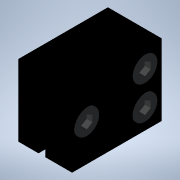
# Autodesk Inventor part: SCHUNK-5503506 Halter fuer NHS KL03
Saved by Autodesk Inventor 2021 (Build 250183000, 183)
## iProperties
Created: 2025-07-30
Part Number: SCHUNK-5503506 Halter fuer NHS KL03
Material: Generic
Catalog Web Link: www.cadenas.de
Description: KLH-bracket
Vendor: SCHUNK
Document SubType Name: Modeling
Designer: psAdmin
Manufacturer: SCHUNK
Mass: 2.81228 g
Surface Area: 23.0408 cm^2
Volume: 2.81228 cm^3
Density: 1 g/cm^3
Appearance: PSOLRGB-35-35-35
Category: PARTsolutions
Company: SCHUNK
Title: SCHUNK-5503506 Halter fuer NHS KL03.
Author: Cadenas PARTsolutions
Comments: bracket
PSOL_IDENT_0: {$CADENAS_DATA/23d-libs/schunk/greifsysteme/greifmodule/greifmodule_pneumatisch/3_finger_zentrischgr
PSOL_IDENT_1: eifer/3_finger_universalgreifer/jgz/jgz_klh.prj},208 {VTYP=3D},{NB=SCHUNK-5503506 Halter fuer NHS KL
PSOL_IDENT_2: 03},{LINA=SCHUNK-5503506 Halter fuer NHS KL03.},{NN=KLH},{DATE=18.12.2024 09:59:27},{GEOMDATE=23.09.
PSOL_IDENT_3: 2021 06:23:09},{VERSION=},{LINEID=10},{WBVAR=},{WBNUMERIC=}  {NB=SCHUNK-5503506 Halter fuer NHS KL03
PSOL_IDENT_4: },{LINA=SCHUNK-5503506 Halter fuer NHS KL03.},{KT=Halter fuer NHS KL03},{IDNR=5503506},{TYP=Halter f
PSOL_IDENT_5: uer NHS KL03},{TYP1=1.000},{L1=2.000},{B=12.000},{T=16.000},{CNSCTN=84799070}
NB: SCHUNK-5503506 Halter fuer NHS KL03
NN: KLH
NT: bracket
NBSYN: SCHUNK-$IDNR. $TYP.
LINA: SCHUNK-5503506 Halter fuer NHS KL03.
CATALOG: SCHUNK
IDNR: 5503506
TYP: Halter fuer NHS KL03
TYP1: 1
L1: 2
B: 12
T: 16
CNSCTN: 84799070
SUPPLIER: SCHUNK
ARTICLENO: SCHUNK-5503506 Halter fuer NHS KL03
BOMINFO: SCHUNK-5503506 Halter fuer NHS KL03.
CREATOR: CADENAS GmbH
Autodesk Inventor part; units mm, degrees
sketch "Skizze_1" plane through (0, 0, 0) normal (0, 1, 0) x (-1, 0, 0)
  line L0 (0, 10) -> (-4.5, 10)
  line L1 (-4.5, 10) -> (-4.5, 3.9686)
  arc A0 (-6, 3.873) -> (-4.5, 3.9686) centre (-5, 0) ccw
  line L2 (-6, 3.873) -> (-6, 10)
  line L3 (-6, 10) -> (-12, 10)
  line L4 (-12, 10) -> (-12, -10)
  line L5 (-12, -10) -> (0, -10)
  line L6 (0, -10) -> (0, 10)
  constraints: 14 end point, 2 point on circle, 1 centre point
extrude "Extrusion1" add sketch "Skizze_1" along normal blind 16
sketch "Sketch2" plane through (12, 0, 10) normal (1, 0, 0) x (0, 0, -1)
  point P0 (16.5, 4.25)
hole "Hole1" at (12, 4.25, -6.5) direction (-1, 0, 0) diameter 6 depth 3.2
sketch "Sketch3" plane through (12, 0, 10) normal (1, 0, 0) x (0, 0, -1)
  point P0 (16.5, 11.75)
hole "Hole2" at (12, 11.75, -6.5) direction (-1, 0, 0) diameter 6 depth 3.2
sketch "Skizze_5" plane through (8.8, 4.25, -6.5) normal (1, 0, 0) x (0, 0, -1)
  circle A0 centre (0, 0) radius 2.75
  constraints: 1 centre point
extrude "Extrusion2" add sketch "Skizze_5" along normal blind 3
sketch "Skizze_6" plane through (11.8, 4.25, -6.5) normal (1, 0, 0) x (0, 0, -1)
  line L0 (-1.25, -0.7217) -> (0, -1.4434)
  line L1 (0, -1.4434) -> (1.25, -0.7217)
  line L2 (1.25, -0.7217) -> (1.25, 0.7217)
  line L3 (1.25, 0.7217) -> (0, 1.4434)
  line L4 (0, 1.4434) -> (-1.25, 0.7217)
  line L5 (-1.25, 0.7217) -> (-1.25, -0.7217)
  constraints: 12 end point
extrude "Extrusion3" cut sketch "Skizze_6" against normal blind 1.3
sketch "Skizze_4" plane through (8.8, 11.75, -6.5) normal (1, 0, 0) x (0, 0, -1)
  circle A0 centre (0, 0) radius 2.75
  constraints: 1 centre point
extrude "Extrusion4" add sketch "Skizze_4" along normal blind 3
sketch "Skizze_7" plane through (11.8, 11.75, -6.5) normal (1, 0, 0) x (0, 0, -1)
  line L0 (-1.25, -0.7217) -> (0, -1.4434)
  line L1 (0, -1.4434) -> (1.25, -0.7217)
  line L2 (1.25, -0.7217) -> (1.25, 0.7217)
  line L3 (1.25, 0.7217) -> (0, 1.4434)
  line L4 (0, 1.4434) -> (-1.25, 0.7217)
  line L5 (-1.25, 0.7217) -> (-1.25, -0.7217)
  constraints: 12 end point
extrude "Extrusion5" cut sketch "Skizze_7" against normal blind 1.3
sketch "Sketch8" plane through (12, 0, 10) normal (1, 0, 0) x (0, 0, -1)
  point P0 (3.5, 8)
hole "Hole3" at (12, 8, 6.5) direction (-1, 0, 0) diameter 6 depth 3.2
sketch "Skizze_12" plane through (8.8, 8, 6.5) normal (1, 0, 0) x (0, 0, -1)
  circle A0 centre (0, 0) radius 2.75
  constraints: 1 centre point
extrude "Extrusion6" add sketch "Skizze_12" along normal blind 3
sketch "Skizze_13" plane through (11.8, 8, 6.5) normal (1, 0, 0) x (0, 0, -1)
  line L0 (-1.25, -0.7217) -> (0, -1.4434)
  line L1 (0, -1.4434) -> (1.25, -0.7217)
  line L2 (1.25, -0.7217) -> (1.25, 0.7217)
  line L3 (1.25, 0.7217) -> (0, 1.4434)
  line L4 (0, 1.4434) -> (-1.25, 0.7217)
  line L5 (-1.25, 0.7217) -> (-1.25, -0.7217)
  constraints: 12 end point
extrude "Extrusion7" cut sketch "Skizze_13" against normal blind 1.3
ref_plane "Naeherungsschalter_Du8_XY" through (5, 0, 0) normal (0, 1, 0) x (1, 0, 0)
ref_plane "Naeherungsschalter_Du8_YZ" through (5, 0, 0) normal (1, 0, 0) x (0, 0, -1)
ref_plane "Naeherungsschalter_Du8_ZX" through (5, 0, 0) normal (0, 0, -1) x (0, 1, 0)
ref_plane "apzbplus_XY" through (4.5, 11.75, -6.5) normal (0, 1, 0) x (1, 0, 0)
ref_plane "apzbplus_YZ" through (4.5, 11.75, -6.5) normal (1, 0, 0) x (0, 0, -1)
ref_plane "apzbplus_ZX" through (4.5, 11.75, -6.5) normal (0, 0, -1) x (0, 1, 0)
ref_plane "jgz64_XY" through (0, 8, 6.5) normal (0, 0, 1) x (1, 0, 0)
ref_plane "jgz64_YZ" through (0, 8, 6.5) normal (1, 0, 0) x (0, 1, 0)
ref_plane "jgz64_ZX" through (0, 8, 6.5) normal (0, 1, 0) x (0, 0, 1)
ref_plane "jpg64_XY" through (0, 11, 0) normal (1, 0, 0) x (0, 0, -1)
ref_plane "jpg64_YZ" through (0, 11, 0) normal (0, 0, -1) x (0, 1, 0)
ref_plane "jpg64_ZX" through (0, 11, 0) normal (0, 1, 0) x (1, 0, 0)
ref_plane "klh1_XY" through (0, 11.75, -6.5) normal (1, 0, 0) x (0, 0, -1)
ref_plane "klh1_YZ" through (0, 11.75, -6.5) normal (0, 0, -1) x (0, 1, 0)
ref_plane "klh1_ZX" through (0, 11.75, -6.5) normal (0, 1, 0) x (1, 0, 0)
ref_plane "klh_64_XY" through (0, 8, -6.5) normal (1, 0, 0) x (0, 0, -1)
ref_plane "klh_64_YZ" through (0, 8, -6.5) normal (0, 0, -1) x (0, 1, 0)
ref_plane "klh_64_ZX" through (0, 8, -6.5) normal (0, 1, 0) x (1, 0, 0)
ref_plane "klh_80_XY" through (0, 4.25, -6.5) normal (1, 0, 0) x (0, 0, -1)
ref_plane "klh_80_YZ" through (0, 4.25, -6.5) normal (0, 0, -1) x (0, 1, 0)
ref_plane "klh_80_ZX" through (0, 4.25, -6.5) normal (0, 1, 0) x (1, 0, 0)
ref_plane "pzn_300_380_XY" through (4.5, 8, 6.5) normal (0, 0, 1) x (1, 0, 0)
ref_plane "pzn_300_380_YZ" through (4.5, 8, 6.5) normal (1, 0, 0) x (0, 1, 0)
ref_plane "pzn_300_380_ZX" through (4.5, 8, 6.5) normal (0, 1, 0) x (0, 0, 1)
ref_plane "vst___geh_XY" through (0, 0, 0) normal (1, 0, 0) x (0, 0, -1)
ref_plane "vst___geh_YZ" through (0, 0, 0) normal (0, 0, -1) x (0, 1, 0)
ref_plane "vst___geh_ZX" through (0, 0, 0) normal (0, 1, 0) x (1, 0, 0)
ref_plane "vst___geh_2_XY" through (0, 16, 0) normal (1, 0, 0) x (0, 0, -1)
ref_plane "vst___geh_2_YZ" through (0, 16, 0) normal (0, 0, -1) x (0, 1, 0)
ref_plane "vst___geh_2_ZX" through (0, 16, 0) normal (0, 1, 0) x (1, 0, 0)
body "Solid1"
